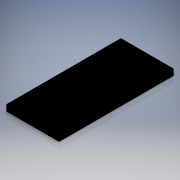
# Autodesk Inventor part: Ceiling Light
Saved by Autodesk Inventor 2018 (Build 220112000, 112)
## iProperties
Created: 2019-11-01
Part Number: Ceiling Light
Material: Generic
Document SubType Name: Modeling
Designer: Jacob
Density: 1 g/cm^3
Appearance: Default
Author: Jacob
Autodesk Inventor part; units mm, degrees
ref_plane "YZ Plane" through (0, 0, 0) normal (1, 0, 0) x (0, 1, 0)
ref_plane "XZ Plane" through (0, 0, 0) normal (0, 1, 0) x (-1, 0, 0)
ref_plane "XY Plane" through (0, 0, 0) normal (0, 0, 1) x (1, 0, 0)
sketch "Sketch1" plane through (0, 0, 0) normal (0, 1, 0) x (-1, 0, 0)
  line L0 (275.463, 597.916) -> (-275.463, 597.916)
  line L1 (-275.463, 597.916) -> (-275.463, -597.916)
  line L2 (-275.463, -597.916) -> (275.463, -597.916)
  line L3 (275.463, -597.916) -> (275.463, 597.916)
  line L4 (275.463, 597.916) -> (-275.463, -597.916) construction
  line L5 (-275.463, 597.916) -> (275.463, -597.916) construction
  point P0 (0, 0)
  dimension "d0" = 1195.832
  dimension "d1" = 550.926
  constraints: 12 end point, 2 midpoint, 2 parallel, 1 horizontal, 1 perpendicular
  measures "d0" distance of L2.end L0.start
  measures "d1" distance of L1.end L2.end
extrude "Extrusion1" add sketch "Sketch1" along normal blind 12.7
sketch "Sketch2" plane through (0, 0, 0) normal (0, -1, 0) x (1, 0, 0)
  line L0 (275.463, 597.916) -> (275.463, -597.916) projected
  line L1 (-275.463, 597.916) -> (275.463, 597.916) projected
  line L2 (-275.463, -597.916) -> (-275.463, 597.916) projected
  line L3 (275.463, -597.916) -> (-275.463, -597.916) projected
  line L4 (272.288, 594.741) -> (-272.288, 594.741)
  line L5 (-272.288, 594.741) -> (-272.288, -594.741)
  line L6 (-272.288, -594.741) -> (272.288, -594.741)
  line L7 (272.288, -594.741) -> (272.288, 594.741)
  line L8 (272.288, 594.741) -> (-272.288, -594.741) construction
  line L9 (-272.288, 594.741) -> (272.288, -594.741) construction
  point P0 (0, 0)
  dimension "d4" = 3.175
  dimension "d5" = 3.175
  constraints: 12 end point, 2 midpoint, 2 parallel, 1 horizontal, 1 perpendicular
  measures "d4" distance between parallel lines of L0 L7
  measures "d5" distance between parallel lines of L4 L1
extrude "Extrusion2" add sketch "Sketch2" along normal blind 50.8
fillet "Fillet1" radius 508 2 edges at (-272.288, 0, 0) (272.288, 0, 0)
sketch "Sketch3" plane through (0, 0, 0) normal (0, -1, 0) x (1, 0, 0)
  line L0 (-275.463, -597.916) -> (275.463, -597.916) projected
  line L1 (50.8, 597.916) -> (-50.8, 597.916)
  line L2 (-50.8, 597.916) -> (-50.8, -597.916)
  line L3 (-50.8, -597.916) -> (50.8, -597.916)
  line L4 (50.8, -597.916) -> (50.8, 597.916)
  line L5 (50.8, 597.916) -> (-50.8, -597.916) construction
  line L6 (-50.8, 597.916) -> (50.8, -597.916) construction
  point P0 (0, 0)
  dimension "d9" = 101.6
  constraints: 12 end point, 2 midpoint, 2 parallel, 1 horizontal, 1 perpendicular, 1 point on line
  measures "d9" distance between parallel lines of L2 L4
extrude "Extrusion3" add sketch "Sketch3" along normal blind 48.26
fillet "Fillet2" radius 50.8 2 edges at (-50.8, -48.26, 0) (50.8, -48.26, 0)
body "Solid1"
